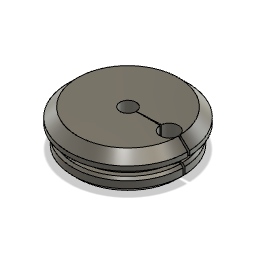
usb grommet v1 (Autodesk Fusion 360 design; units mm, degrees)
Autodesk Fusion 360 part; units mm, degrees
sketch "Sketch1" plane through (0, 0, 0) normal (0, 0, 1) x (1, 0, 0)
  line L0 (0, 0) -> (94.4785, 0) construction
  line L1 (10.5, 0) -> (10.5, -2)
  line L2 (10.5, -2) -> (12, -2)
  line L3 (12, -2) -> (12, -5)
  line L4 (12, -5) -> (1.75, -5)
  line L5 (1.75, -5) -> (1.75, 3)
  line L6 (12, 0) -> (10.5, 0)
  line L7 (12, 0) -> (13, 0)
  line L8 (13, 0) -> (13, 3)
  line L9 (1.75, 3) -> (13, 3)
  dimension "d1" = 2
  dimension "d4" = 10.5
  dimension "d5" = 1.5
  dimension "d6" = 3
  dimension "d7" = 8
  dimension "d8" = 1.75
  dimension "d9" = 1
  dimension "d10" = 11.25
  constraint coincident L0.start origin
  constraint horizontal L0
  constraint coincident L0 L1.start
  constraint perpendicular L0 L1
  constraint perpendicular L1 L2
  constraint perpendicular L2 L3
  constraint perpendicular L1 L4
  constraint perpendicular L0 L5
  constraint coincident L0 L6.start
  constraint parallel L0 L7
  constraint perpendicular L7 L8
  constraint perpendicular L8 L9
  measures "d1" distance of L1.start L1.end
  measures "d4" distance of L0.start L1
  measures "d5" distance of L1.end L2.end
  measures "d6" distance of L2.end L3.end
  measures "d7" distance of L4.end L5.end
  measures "d8" distance of L0.start L5
  measures "d9" distance of L6.start L7.end
  measures "d10" distance of L5 L8
revolve "Revolve1" add sketch "Sketch1" angle 358 about axis through (0, 1.75, 0) along (0, -1, 0)
chamfer "Chamfer1" distance 2 angle 45 1 edges at (-12.998, 3, 0.2269)
chamfer "Chamfer2" distance 1 angle 45 1 edges at (-11.9982, -5, 0.2094)
sketch "Sketch2" plane through (0, 3, 0) normal (0, 1, 0) x (-1, 0, 0)
  line L0 (-11, 0) -> (-1.75, 0)
  arc A0 (-1.7489, -0.0611) -> (-1.75, 0) centre (0, 0) ccw
  line L1 (-1.7489, -0.0611) -> (-10.9933, -0.3839)
  line L2 (0, 0) -> (-17.3429, 0.0305) construction
  circle A1 centre (-9, 0) radius 2
  line L3 (-10.5, 0) -> (-13, 0)
  arc A2 (-12.9921, -0.4537) -> (-13, 0) centre (0, 0) ccw
  line L4 (-12.9921, -0.4537) -> (-10.4936, -0.3664)
  arc A3 (-10.4936, -0.3664) -> (-10.5, 0) centre (0, 0) ccw
  arc A4 (-10.9933, -0.3839) -> (-11, 0) centre (0, 0) ccw
  dimension "d14" = 4
  dimension "d15" = 1.5
  constraint coincident A0.centre L2.start
  constraint coincident L0 A1.centre
  measures "d14" diameter of A1
  measures "d15" distance of A1.centre L3.start
extrude "Extrude1" cut sketch "Sketch2" against normal blind 20 contours L0 A1 L3 A3 | L0 L1 A1 L3 L4 | L0 A1 A3 | L1 A1 L4 A3 | L1 A1 A3
chamfer "Chamfer3" distance 0.5 angle 45 1 edges at (-11.9982, -2, 0.2094)
equation "d4 = ( 21 / 2 ) * 1 mm"
equation "d8 = ( 3.5 / 2 ) * 1 mm"
named bodies: "USB grommet"
